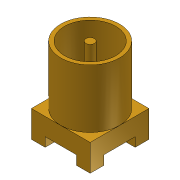
# Autodesk Inventor part: MOLEX 73415-2061
Saved by Autodesk Inventor 2014 SP1 (Build 180222100, 222)
## iProperties
Created: 2012-11-10
Part Number: MOLEX 73415-2061
Document SubType Name: Modeling
Designer: Robert Davis
Density: 8.47 g/cm^3
Material: Brass, Soft Yellow
Mass: 0.0287956 g
Surface Area: 0.307064 cm^2
Volume: 0.00339971 cm^3
Description: MMCX JACK, 50 OHM SMD
Appearance: Brass - Satin
Author: Robert Davis
Autodesk Inventor part; units mm, degrees
ref_plane "YZ Plane" through (0, 0, 0) normal (1, 0, 0) x (0, 1, 0)
ref_plane "XZ Plane" through (0, 0, 0) normal (0, 1, 0) x (-1, 0, 0)
sketch "Sketch1" plane through (0, 0, 0) normal (0, 0, 1) x (1, 0, 0)
  line L0 (0, 0) -> (0.4099, 0)
  line L1 (0, 0) -> (0, 0.6993)
  circle A0 centre (0, 0) radius 0.355
  line L2 (-1.725, 1.725) -> (1.725, 1.725) construction
  line L3 (1.725, 1.725) -> (1.725, -1.725) construction
  line L4 (1.725, -1.725) -> (-1.725, -1.725) construction
  line L5 (-1.725, -1.725) -> (-1.725, 1.725) construction
  line L6 (-1.725, 1.725) -> (-0.915, 1.725)
  line L7 (-0.915, 1.725) -> (-0.915, 0.915)
  line L8 (-0.915, 0.915) -> (-1.725, 0.915)
  line L9 (-1.725, 0.915) -> (-1.725, 1.725)
  line L10 (-1.725, -1.725) -> (-0.915, -1.725)
  line L11 (-0.915, -1.725) -> (-0.915, -0.915)
  line L12 (-0.915, -0.915) -> (-1.725, -0.915)
  line L13 (-1.725, -0.915) -> (-1.725, -1.725)
  line L14 (1.725, -1.725) -> (0.915, -1.725)
  line L15 (0.915, -1.725) -> (0.915, -0.915)
  line L16 (0.915, -0.915) -> (1.725, -0.915)
  line L17 (1.725, -0.915) -> (1.725, -1.725)
  line L18 (1.725, 1.725) -> (0.915, 1.725)
  line L19 (0.915, 1.725) -> (0.915, 0.915)
  line L20 (0.915, 0.915) -> (1.725, 0.915)
  line L21 (1.725, 0.915) -> (1.725, 1.725)
  dimension "d25" = 3.45
  dimension "d26" = 3.45
  dimension "d27" = 0.81
  dimension "d28" = 0.71
  constraints: 44 end point, 10 horizontal, 10 vertical, 7 equal length, 1 centre point, 1 coincident, 2 other
  measures "d25" distance of L2.start L2.end
  measures "d26" distance of L2.end L3.end
  measures "d27" distance of L8.end L2.start
  measures "d28" diameter of A0
extrude "Extrusion1" add sketch "Sketch1" along normal blind 0.54
ref_plane "Work Plane2" through (0, 0, 0.54) normal (0, 0, 1) x (1, 0, 0)
sketch "Sketch2" plane through (0, 0, 0.54) normal (0, 0, 1) x (1, 0, 0)
  line L0 (-1.725, 1.725) -> (1.725, 1.725)
  line L1 (1.725, 1.725) -> (1.725, -1.725)
  line L2 (1.725, -1.725) -> (-1.725, -1.725)
  line L3 (-1.725, -1.725) -> (-1.725, 1.725)
  line L4 (0, 0) -> (0.4406, 0)
  line L5 (0, 0) -> (0, 0.4944)
  constraints: 12 end point, 5 coincident, 2 horizontal, 2 vertical, 2 other
extrude "Extrusion2" add sketch "Sketch2" along normal blind 1.03
sketch "Sketch3" plane through (0, 0, 1.57) normal (0, 0, 1) x (1, 0, 0)
  circle A0 centre (0, 0) radius 1.725
  circle A1 centre (0, 0) radius 1.5
  circle A2 centre (0, 0) radius 0.25
  dimension "d20" = 0.5
  dimension "d21" = 3.45
  dimension "d22" = 3
  constraints: 3 centre point
  measures "d20" diameter of A2
  measures "d21" diameter of A0
  measures "d22" diameter of A1
extrude "Extrusion3" add sketch "Sketch3" along normal blind 3.43
body "Solid1"
